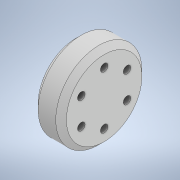
# Autodesk Inventor part: 711136
Saved by Autodesk Inventor 2022 (Build 260153000, 153)
## iProperties
Created: 2021-10-22
Part Number: 711136
Material: Типовые
Document SubType Name: Modeling
Designer: RaNSiD
Density: 1 g/cm^3
Appearance: По умолчанию
Author: RaNSiD
Autodesk Inventor part; units mm, degrees
ref_plane "YZ Plane" through (0, 0, 0) normal (1, 0, 0) x (0, 1, 0)
ref_plane "XZ Plane" through (0, 0, 0) normal (0, 1, 0) x (-1, 0, 0)
ref_plane "XY Plane" through (0, 0, 0) normal (0, 0, 1) x (1, 0, 0)
sketch "Эскиз1" plane through (0, 0, 0) normal (0, 0, 1) x (1, 0, 0)
  line L0 (0, 0) -> (0, 20)
  line L1 (0, 20) -> (2.8284, 22.8284)
  line L2 (0, 0) -> (15, 0)
  line L3 (15, 0) -> (15, 20)
  line L4 (15, 20) -> (12.1716, 22.8284)
  line L5 (12.1716, 22.8284) -> (2.8284, 22.8284)
  dimension "d0" = 20
  dimension "d1" = 4
  dimension "d2" = 135
  dimension "d3" = 15
  dimension "d4" = 4
  dimension "d5" = 135
  constraints: 12 end point, 1 horizontal, 1 parallel, 1 perpendicular, 1 vertical
  measures "d0" distance of L0.start L0.end
  measures "d1" distance of L0.end L1.end
  measures "d2" angle of L0 L1
  measures "d3" distance of L0.start L2.end
  measures "d4" distance of L3.end L4.end
  measures "d5" angle of L4 L3
revolve "Вращение1" add sketch "Эскиз1" angle 360 about axis through (0, 0, 0) along (1, 0, 0)
sketch "Эскиз2" plane through (0, 0, 0) normal (-1, 0, 0) x (0, 0, 1)
  point P0 (0, 0)
  point P1 (0, 18)
  point P2 (-15.5885, 9)
  point P3 (-15.5885, -9)
  point P4 (0, -18)
  point P5 (15.5885, -9)
  point P6 (15.5885, 9)
  dimension "d7" = 18
  dimension "d10" = 360
  constraints: 1 vertical alignment, 7 other
  measures "d7" distance of point (0, 0) point (0, 18)
hole "Отверстие1" at (0, 18, 0) at (0, 9, -15.5885) at (0, -9, -15.5885) at (0, -18, 0) at (0, -9, 15.5885) at (0, 9, 15.5885) direction (1, 0, 0) diameter 4 depth 4
sketch "Эскиз3" plane through (15, 0, 0) normal (1, 0, 0) x (0, 0, -1)
  point P0 (0, 0)
  point P1 (0, 14)
  point P2 (-12.1244, 7)
  point P3 (-12.1244, -7)
  point P4 (0, -14)
  point P5 (12.1244, -7)
  point P6 (12.1244, 7)
  dimension "d19" = 14
  dimension "d22" = 360
  constraints: 1 vertical alignment, 7 other
  measures "d19" distance of point (0, 0) point (0, 14)
hole "Отверстие2" at (15, 14, 0) at (15, 7, 12.1244) at (15, -7, 12.1244) at (15, -14, 0) at (15, -7, -12.1244) at (15, 7, -12.1244) direction (-1, 0, 0) diameter 4 depth 4 tip angle 118
sketch "Эскиз4" plane through (0, 0, 0) normal (0, 0, 1) x (1, 0, 0)
  line L0 (0, 0) -> (0, 8)
  line L1 (0, -10) -> (0, 10) projected
  line L2 (0, 8) -> (0.7, 7.3)
  line L3 (0, 8) -> (0.9899, 8) construction
  line L4 (0.7, 7.3) -> (6.643, 7.3)
  line L5 (6.643, 7.3) -> (6.643, 8)
  line L6 (6.643, 8) -> (7.343, 8)
  line L7 (7.343, 8) -> (7.343, 7.3)
  line L8 (7.343, 7.3) -> (10, 0)
  line L9 (10, 0) -> (0, 0)
  dimension "d31" = 45
  dimension "d32" = 70
  dimension "d33" = 8
  dimension "d35" = 0.7
  dimension "d36" = 0.7
  dimension "d37" = 10
  constraints: 18 end point, 5 perpendicular, 2 point on line, 1 equal length, 1 horizontal, 1 horizontal alignment
  measures "d31" angle of L2 L3
  measures "d32" angle of L9 L8
  measures "d33" distance of L0.start L0.end
  measures "d35" distance of L6.end L7.end
  measures "d36" distance of L5.end L6.end
  measures "d37" distance of L8.end L0.start
revolve "Вращение2" cut sketch "Эскиз4" angle 360 about axis through (10, 0, 0) along (-1, 0, 0)
thread "Резьба1" size "M15x1.5" class "6H" standard "ANSI Metric M Profile" full length
thread "Резьба2" size "Rc 1/16" standard "ISO Taper Internal" full length
